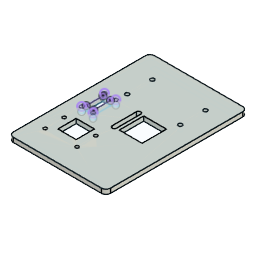
LID (Autodesk Fusion 360 design; units mm, degrees)
part number: 2026-04-01-18-16-49-366
Autodesk Fusion 360 part; units mm, degrees
sketch "Sketch5" plane through (0, 0, 0) normal (0, 0, 1) x (1, 0, 0)
  line L0 (3, 0) -> (61, 0)
  line L1 (64, 3) -> (64, 90)
  line L2 (61, 93) -> (3, 93)
  line L3 (0, 90) -> (0, 3)
  arc A0 (0, 3) -> (3, 0) centre (3, 3) ccw
  arc A1 (3, 93) -> (0, 90) centre (3, 90) ccw
  arc A2 (64, 90) -> (61, 93) centre (61, 90) ccw
  arc A3 (61, 0) -> (64, 3) centre (61, 3) ccw
  point P0 (64, 0)
  point P1 (0, 93)
  dimension "d27" = 64
  dimension "d28" = 93
  dimension "d29" = 3
  constraint horizontal L0
  constraint vertical L1
  constraint horizontal L2
  constraint vertical L3
  constraint coincident origin L0
  constraint coincident origin L3
  constraint tangent L0 A0
  constraint tangent L3 A0
  constraint coincident P1 L2
  constraint coincident P1 L3
  constraint tangent L2 A1
  constraint tangent L3 A1
  constraint equal A0 A1
  constraint tangent L1 A2
  constraint tangent L2 A2
  constraint equal A0 A2
  constraint coincident P0 L0
  constraint coincident P0 L1
  constraint tangent L0 A3
  constraint tangent L1 A3
  constraint equal A0 A3
  measures "d27" distance of origin P0
  measures "d28" distance of origin P1
  measures "d29" radius of A0
extrude "Extrude5" add sketch "Sketch5" along normal blind 3
sketch "Sketch6" plane through (0, 0, 0) normal (0, 0, -1) x (1, 0, 0)
  arc A0 (64, -3) -> (61, 0) centre (61, -3) ccw
  line L0 (61, 0) -> (3, 0)
  arc A1 (3, 0) -> (0, -3) centre (3, -3) ccw
  line L1 (0, -3) -> (0, -90)
  arc A2 (0, -90) -> (3, -93) centre (3, -90) ccw
  line L2 (3, -93) -> (61, -93)
  arc A3 (61, -93) -> (64, -90) centre (61, -90) ccw
  line L3 (64, -90) -> (64, -3)
  line L4 (3, -3) -> (61, -3)
  line L5 (61, -3) -> (61, -90)
  line L6 (61, -90) -> (3, -90)
  line L7 (3, -90) -> (3, -3)
  line L8 (6, -3) -> (58, -3)
  line L9 (58, -3) -> (58, -6)
  line L10 (58, -6) -> (6, -6)
  line L11 (6, -6) -> (6, -3)
  line L12 (6, -90) -> (58, -90)
  line L13 (58, -90) -> (58, -87)
  line L14 (58, -87) -> (6, -87)
  line L15 (6, -87) -> (6, -90)
  dimension "d32" = 58
  dimension "d33" = 87
  dimension "d34" = 3
  dimension "d35" = 3
  dimension "d36" = 52
  dimension "d37" = 3
  dimension "d38" = 3
  dimension "d39" = 52
  dimension "d40" = 3
  constraint horizontal L4
  constraint vertical L5
  constraint horizontal L6
  constraint vertical L7
  constraint horizontal L8
  constraint vertical L9
  constraint horizontal L10
  constraint vertical L11
  constraint coincident L4 L8.start
  constraint horizontal L12
  constraint vertical L13
  constraint horizontal L14
  constraint vertical L15
  constraint coincident L6 L12.start
  measures "d32" distance of A1.centre A0.centre
  measures "d33" distance of A1.centre A2.centre
  measures "d34" distance of L1 L7
  measures "d35" distance of L0 L4
  measures "d36" distance of L8.start L8.end
  measures "d37" distance of L8.start L10.end
  measures "d38" distance of L7 L11
  measures "d39" distance of L12.start L12.end
  measures "d40" distance of L12.start L14.end
extrude "Extrude6" add sketch "Sketch6" along normal blind 4 contours L4 L8 L9 L10 L11 | L6 L12 L13 L14 L15
sketch "Sketch8" plane through (0, 0, 0) normal (0, 0, -1) x (1, 0, 0)
  line L0 (6, -6) -> (6, -3)
  line L1 (6, -3) -> (58, -3)
  line L2 (58, -3) -> (58, -6)
  line L3 (58, -6) -> (6, -6)
  line L4 (6, -87) -> (58, -87)
  line L5 (58, -87) -> (58, -90)
  line L6 (58, -90) -> (6, -90)
  line L7 (6, -90) -> (6, -87)
  arc A0 (64, -3) -> (61, 0) centre (61, -3) ccw
  line L8 (61, 0) -> (3, 0)
  arc A1 (3, 0) -> (0, -3) centre (3, -3) ccw
  line L9 (0, -3) -> (0, -90)
  arc A2 (0, -90) -> (3, -93) centre (3, -90) ccw
  line L10 (3, -93) -> (61, -93)
  arc A3 (61, -93) -> (64, -90) centre (61, -90) ccw
  line L11 (64, -90) -> (64, -3)
  circle A4 centre (15.94, -61.99) radius 1.27
  circle A5 centre (15.94, -78.61) radius 1.27
  circle A6 centre (50.9, -78.61) radius 1.27
  circle A7 centre (50.9, -61.99) radius 1.27
  line L12 (64, -81) -> (0, -81)
  line L13 (0, -81) -> (0, -59.6)
  line L14 (0, -59.6) -> (64, -59.6)
  line L15 (64, -59.6) -> (64, -81)
  dimension "d52" = 2.54
  dimension "d55" = 2.54
  dimension "d58" = 2.54
  dimension "d61" = 2.54
  dimension "d85" = 64
  dimension "d86" = 21.4
  dimension "d87" = 6
  dimension "d92" = 2.39
  dimension "d93" = 2.39
  dimension "d96" = 2.39
  dimension "d97" = 15.94
  dimension "d98" = 2.39
  dimension "d99" = 15.94
  dimension "d100" = 50.9
  dimension "d101" = 50.9
  constraint horizontal L12
  constraint vertical L13
  constraint horizontal L14
  constraint vertical L15
  constraint coincident L11 L12.start
  measures "d52" diameter of A4
  measures "d55" diameter of A5
  measures "d58" diameter of A6
  measures "d61" diameter of A7
  measures "d85" distance of L12.start L12.end
  measures "d86" distance of L12.start L14.end
  measures "d87" distance of L4 L12
  measures "d92" distance of A7.centre L14
  measures "d93" distance of A6.centre L12
  measures "d96" distance of A5.centre L12
  measures "d97" distance of A5.centre L13
  measures "d98" distance of A4.centre L14
  measures "d99" distance of A4.centre L13
  measures "d100" distance of A6.centre L13
  measures "d101" distance of A7.centre L13
extrude "Extrude8" cut sketch "Sketch8" against normal blind 3 contours A4 | A5 | A6 | A7
sketch "Sketch9" plane through (0, 0, 0) normal (0, 0, -1) x (1, 0, 0)
  circle A0 centre (50.9, -61.99) radius 1.27
  circle A1 centre (50.9, -78.61) radius 1.27
  circle A2 centre (15.94, -61.99) radius 1.27
  circle A3 centre (15.94, -78.61) radius 1.27
  line L0 (6, -6) -> (6, -3)
  line L1 (6, -3) -> (58, -3)
  line L2 (58, -3) -> (58, -6)
  line L3 (58, -6) -> (6, -6)
  line L4 (6, -87) -> (58, -87)
  line L5 (58, -87) -> (58, -90)
  line L6 (58, -90) -> (6, -90)
  line L7 (6, -90) -> (6, -87)
  arc A4 (64, -3) -> (61, 0) centre (61, -3) ccw
  line L8 (61, 0) -> (3, 0)
  arc A5 (3, 0) -> (0, -3) centre (3, -3) ccw
  line L9 (0, -3) -> (0, -90)
  arc A6 (0, -90) -> (3, -93) centre (3, -90) ccw
  line L10 (3, -93) -> (61, -93)
  arc A7 (61, -93) -> (64, -90) centre (61, -90) ccw
  line L11 (64, -90) -> (64, -3)
  circle A8 centre (8, -40) radius 1.27
  circle A9 centre (8, -55) radius 1.27
  circle A10 centre (15.5, -40) radius 1.27
  circle A11 centre (15.5, -55) radius 1.27
  line L12 (9, -42) -> (14, -42)
  line L13 (14, -42) -> (14, -53)
  line L14 (14, -53) -> (9, -53)
  line L15 (9, -53) -> (9, -42)
  dimension "d70" = 2.54
  dimension "d73" = 2.54
  dimension "d76" = 2.54
  dimension "d79" = 2.54
  constraint horizontal L12
  constraint vertical L13
  constraint horizontal L14
  constraint vertical L15
  measures "d70" diameter of A8
  measures "d73" diameter of A9
  measures "d76" diameter of A10
  measures "d79" diameter of A11
extrude "Extrude9" cut sketch "Sketch9" against normal blind 3 contours A8 | A9 | A10 | A11 | L12 L13 L14 L15
fillet "Fillet5" radius 1.5 4 edges at (32, 3, -4) (32, 6, -4) (32, 87, -4) (32, 90, -4)
sketch "Sketch11" plane through (0, 0, 3) normal (0, 0, 1) x (-1, 0, 0)
  circle A0 centre (-50.9, -61.99) radius 1.27
  circle A1 centre (-50.9, -78.61) radius 1.27
  circle A2 centre (-15.94, -61.99) radius 1.27
  circle A3 centre (-15.94, -78.61) radius 1.27
  arc A4 (-61, 0) -> (-64, -3) centre (-61, -3) ccw
  line L0 (-64, -3) -> (-64, -90)
  arc A5 (-64, -90) -> (-61, -93) centre (-61, -90) ccw
  line L1 (-61, -93) -> (-3, -93)
  arc A6 (-3, -93) -> (0, -90) centre (-3, -90) ccw
  line L2 (0, -90) -> (0, -3)
  arc A7 (0, -3) -> (-3, 0) centre (-3, -3) ccw
  line L3 (-3, 0) -> (-61, 0)
  line L4 (-14, -53) -> (-14, -42)
  line L5 (-14, -42) -> (-9, -42)
  line L6 (-9, -42) -> (-9, -53)
  line L7 (-9, -53) -> (-14, -53)
  circle A8 centre (-15.5, -40) radius 1.27
  circle A9 centre (-8, -55) radius 1.27
  circle A10 centre (-8, -40) radius 1.27
  circle A11 centre (-15.5, -55) radius 1.27
sketch "Sketch12" plane through (0, 0, 3) normal (0, 0, 1) x (-1, 0, 0)
  line L0 (-6.497, -13.503) -> (-6.497, -37.303)
  line L1 (-6.497, -37.303) -> (-31.497, -37.303)
  line L2 (-31.497, -37.303) -> (-31.497, -13.503)
  line L3 (-31.497, -13.503) -> (-6.497, -13.503)
  circle A0 centre (-8.497, -15.503) radius 1.1
  circle A1 centre (-29.497, -15.503) radius 1.1
  circle A2 centre (-8.497, -28.003) radius 1.1
  circle A3 centre (-29.297, -28.003) radius 1.1
  line L4 (-12.997, -19.403) -> (-12.997, -31.403)
  line L5 (-12.997, -31.403) -> (-24.997, -31.403)
  line L6 (-24.997, -31.403) -> (-24.997, -19.403)
  line L7 (-24.997, -19.403) -> (-12.997, -19.403)
  dimension "d106" = 23.8
  dimension "d107" = 25
  dimension "d108" = 2.2
  dimension "d109" = 2
  dimension "d110" = 2
  dimension "d111" = 2.2
  dimension "d112" = 2
  dimension "d113" = 2
  dimension "d114" = 2.2
  dimension "d115" = 2
  dimension "d116" = 14.5
  dimension "d117" = 2.2
  dimension "d118" = 2.2
  dimension "d119" = 14.5
  dimension "d120" = 12
  dimension "d121" = 12
  dimension "d122" = 6.5
  dimension "d123" = 5.9
  measures "d106" distance of L0.start L0.end
  measures "d107" distance of L0.start L2.end
  measures "d108" diameter of A0
  measures "d109" distance of L0 A0.centre
  measures "d110" distance of L3 A0.centre
  measures "d111" diameter of A1
  measures "d112" distance of L3 A1.centre
  measures "d113" distance of L2 A1.centre
  measures "d114" diameter of A2
  measures "d115" distance of L0 A2.centre
  measures "d116" distance of L3 A2.centre
  measures "d117" diameter of A3
  measures "d118" distance of L2 A3.centre
  measures "d119" distance of L3 A3.centre
  measures "d120" distance of L4.start L4.end
  measures "d121" distance of L4.start L6.end
  measures "d122" distance of L0 L4
  measures "d123" distance of L1 L5
extrude "Extrude10" cut sketch "Sketch12" against normal blind 3 contours A0 | A1 | A2 | A3 | L4 L5 L6 L7
sketch "Sketch13" plane through (0, 0, 3) normal (0, 0, 1) x (-1, 0, 0)
  line L0 (-29, -55.0268) -> (-31.8, -55.0268)
  line L1 (-31.8, -55.0268) -> (-31.8, -39.0268)
  line L2 (-31.8, -39.0268) -> (-29, -39.0268)
  line L3 (-29, -39.0268) -> (-29, -55.0268)
  arc A0 (-31.8, -55.0268) -> (-29, -55.0268) centre (-30.4, -55.0268) ccw
  arc A1 (-29, -39.0268) -> (-31.8, -39.0268) centre (-30.4, -39.0268) ccw
  line L4 (-33.8, -55) -> (-48.8, -55)
  line L5 (-48.8, -55) -> (-48.8, -39)
  line L6 (-48.8, -39) -> (-33.8, -39)
  line L7 (-33.8, -39) -> (-33.8, -55)
  line L8 (-14, -42) -> (-14, -53)
  dimension "d126" = 2.8
  dimension "d127" = 16
  dimension "d128" = 15
  dimension "d129" = 16
  dimension "d130" = 2
  dimension "d133" = 15
  constraint horizontal L0
  constraint vertical L1
  constraint horizontal L2
  constraint vertical L3
  constraint tangent L1 A0
  constraint tangent L1 A1
  constraint horizontal L4
  constraint vertical L5
  constraint horizontal L6
  constraint vertical L7
  measures "d126" distance of L0.start L0.end
  measures "d127" distance of L0.start L2.end
  measures "d128" distance of L4.start L4.end
  measures "d129" distance of L4.start L6.end
  measures "d130" distance of L1 L7
  measures "d133" distance of L3 L8
extrude "Extrude11" cut sketch "Sketch13" against normal blind 3
